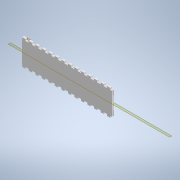
# Autodesk Inventor part: 00_Baseplate_Simmo_side3
Saved by Autodesk Inventor 2022 (Build 260153000, 153)
## iProperties
Created: 2022-04-28
Part Number: 00_Baseplate_Simmo_side3
Material: Generisch
Document SubType Name: Modeling
Designer: diederichbenedict
Density: 1 g/cm^3
Appearance: Vorgabe
Author: diederichbenedict
Autodesk Inventor part; units mm, degrees
ref_plane "YZ Plane" through (0, 0, 0) normal (1, 0, 0) x (0, 1, 0)
ref_plane "XZ Plane" through (0, 0, 0) normal (0, 1, 0) x (-1, 0, 0)
ref_plane "XY Plane" through (0, 0, 0) normal (0, 0, 1) x (1, 0, 0)
ref_plane "Arbeitsebene1" through (0, 0, 0) normal (0, 0, 1) x (1, 0, 0)
sketch "Skizze1" plane through (0, 0, 0) normal (0, 0, 1) x (1, 0, 0)
  line L0 (0, 5) -> (10, 5) projected
  line L1 (10, 0) -> (0, 0) projected
  line L2 (10, 0) -> (10, 5) projected
  line L3 (442.7944, 5) -> (442.7944, 0) projected
  line L4 (0, -68) -> (10, -68) projected
  line L5 (0, 5) -> (295.8, 5)
  line L6 (295.8, 5) -> (295.8, -68)
  line L7 (295.8, -68) -> (0, -68)
  line L8 (0, -68) -> (0, 5)
  line L9 (0, -68) -> (295.8, -68)
  line L10 (295.8, -68) -> (295.8, -74)
  line L11 (295.8, -74) -> (0, -74)
  line L12 (0, -74) -> (0, -68)
  line L13 (0, 0) -> (0, 5) projected
  line L14 (255.9, -69) -> (255.9, -74)
  line L15 (295.8, 6) -> (295.8, 1)
  point P0 (450, -68)
  point P1 (450, 0)
  point P2 (442.7944, 5)
  point P3 (450, -68)
  dimension "d0" = 6
  dimension "d29" = 0
  constraints: 20 end point, 4 parallel, 2 horizontal, 2 perpendicular, 2 vertical, 4 other
  measures "d0" distance of L6.end L10.end
  measures "d29" distance between parallel lines of L15 L6
extrude "Extrusion1" add sketch "Skizze1" along normal blind 6
sketch "Skizze2" plane through (0, 0, 0) normal (0, 0, -1) x (1, 0, 0)
  line L0 (20, 0) -> (20, -5) projected
  line L1 (10, -5) -> (10, 0) projected
  line L2 (0, -5) -> (0, 74) projected
  line L3 (9.8, -5) -> (20.2, -5)
  line L4 (20.2, -5) -> (20.2, 0)
  line L5 (20.2, 0) -> (9.8, 0)
  line L6 (9.8, 0) -> (9.8, -5)
  point P0 (0, 0)
  dimension "d6" = 0
  dimension "d17" = 0.2
  dimension "d18" = 0.2
  constraints: 8 end point, 2 parallel, 1 horizontal, 1 perpendicular
  measures "d6" distance from line of L1.end L5
  measures "d17" distance between parallel lines of L4 L0
  measures "d18" distance between parallel lines of L6 L1
extrude "Extrusion2" cut sketch "Skizze2" against normal blind 6
sketch "Skizze3" plane through (20.2, 5, 0) normal (0, 1, 0) x (1, 0, 0)
  line L0 (275.6, 0) -> (0, 0) projected
  line L1 (-10.4, -6) -> (0, -6) projected
  line L2 (0, 0) -> (0, -6) projected
  circle A0 centre (-5.2, -3) radius 1.5
  line L3 (-10.4, -6) -> (-10.4, 0) projected
  point P0 (-20.2, 0)
  point P1 (4.8, 3)
  point P2 (429.8, 0)
  point P3 (429.8, -6)
  dimension "d16" = 3
  dimension "d19" = 5.2
  constraints: 1 centre point
  measures "d16" diameter of A0
  measures "d19" distance from line of A0.centre L3
hole "Bohrung1" at (15, 5, 3) direction (0, -1, 0) diameter 3 depth 20
pattern_linear "Rechteckige Anordnung1" count 24 spacing 20 along (1, 0, 0) of "Extrusion2", "Bohrung1"
ref_plane "Arbeitsebene2" through (0, -34.5, 0) normal (0, -1, 0) x (1, 0, 0)
mirror "Spiegeln1" about plane through (0, -34.5, 0) normal (0, -1, 0) of "Extrusion2", "Bohrung1", "Rechteckige Anordnung1"
sketch "Skizze4" plane through (0, 5, 6) normal (0, 1, 0) x (1, 0, 0)
  line L0 (9.8, 0) -> (0, 0) projected
  line L1 (19.9969, 0) -> (-5.9169, 0)
  line L2 (-5.9169, 0) -> (-5.9169, 6)
  line L3 (-5.9169, 6) -> (19.9969, 6)
  line L4 (19.9969, 6) -> (19.9969, 0)
  line L5 (0, 6) -> (0, 0) projected
  line L6 (9.8, 0) -> (9.8, 6) projected
  line L7 (19.9, 6) -> (19.9, 0)
  point P0 (3.75, 0)
  point P1 (0, 0)
  point P2 (0, 6)
  constraints: 10 end point, 2 parallel, 1 horizontal, 1 perpendicular, 1 point on line, 1 vertical, 2 other
extrude "Extrusion3" cut sketch "Skizze4" against normal through all
